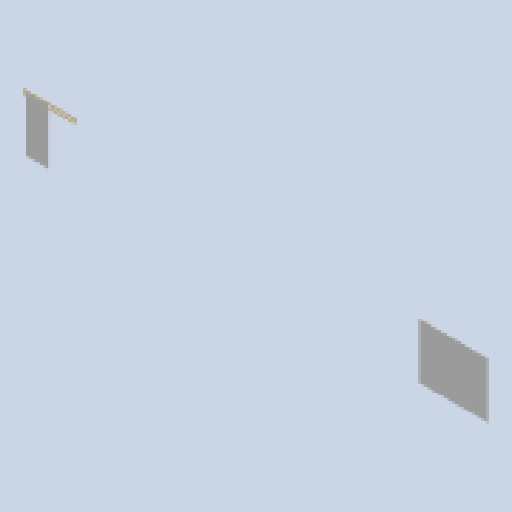
# Autodesk Inventor part: пол1
Saved by Autodesk Inventor 2024.2 (Build 282272000, 272)
## iProperties
Created: 2025-11-16
Part Number: пол1
Material: Типовые
Document SubType Name: Modeling
Designer: katya_notebook
Density: 1 g/cm^3
Appearance: По умолчанию
Author: katya_notebook
Autodesk Inventor part; units mm, degrees
ref_plane "YZ Plane" through (0, 0, 0) normal (1, 0, 0) x (0, 1, 0)
ref_plane "XZ Plane" through (0, 0, 0) normal (0, 1, 0) x (-1, 0, 0)
ref_plane "XY Plane" through (0, 0, 0) normal (0, 0, 1) x (1, 0, 0)
ref_plane "РабПлоскость1" through (0, 0, 0) normal (0, 0, 1) x (1, 0, 0)
sketch "Эскиз1" plane through (0, 0, 0) normal (0, 0, 1) x (1, 0, 0)
  line L0 (0, 0) -> (0, 16) projected
  line L1 (0, 16) -> (201.062, 16) projected
  line L2 (0, 16) -> (100, 16)
  line L3 (100, 16) -> (100, -226)
  line L4 (100, -226) -> (0, -226)
  line L5 (0, -226) -> (0, 16)
  line L6 (2010.62, 0) -> (2010.62, 16) projected
  line L7 (1809.558, 16) -> (2010.62, 16) projected
  line L8 (2010.62, 16) -> (1710.62, 16)
  line L9 (1710.62, 16) -> (1710.62, -226)
  line L10 (1710.62, -226) -> (2010.62, -226)
  line L11 (2010.62, -226) -> (2010.62, 16)
  dimension "d0" = 242
  dimension "d1" = 100
  dimension "d2" = 242
  dimension "d3" = 300
  constraints: 16 end point, 4 parallel, 2 horizontal, 2 perpendicular
  measures "d0" distance of L4.end L0.end
  measures "d1" distance of L3.end L4.end
  measures "d2" distance of L10.end L6.end
  measures "d3" distance of L9.end L10.end
extrude "Выдавливание1" add sketch "Эскиз1" along normal blind 3
